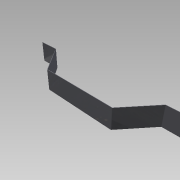
# Autodesk Inventor part: handle
Saved by Autodesk Inventor 2012 (Build 160160000, 160)
## iProperties
Created: 2012-04-18
Part Number: handle
Material: Default
Document SubType Name: Sheet Metal
Designer: thanos
Density: 1 g/cm^3
Sheet Metal Rule: Default_mm
Mass: 50.8146 g
Surface Area: 530.472 cm^2
Volume: 50.8146 cm^3
Author: thanos
Autodesk Inventor part; units mm, degrees
note: some values were not read from the file. Chosen so that the rebuilt part matches the saved one: flange form of "Plate1".
ref_plane "YZ Plane" through (0, 0, 0) normal (1, 0, 0) x (0, 1, 0)
ref_plane "XZ Plane" through (0, 0, 0) normal (0, 1, 0) x (-1, 0, 0)
ref_plane "XY Plane" through (0, 0, 0) normal (0, 0, 1) x (1, 0, 0)
sketch "Sketch3" plane through (0, 0, 0) normal (0, 0, 1) x (1, 0, 0)
  line L0 (-156.4592, 62.5093) -> (-106.4592, 62.5093)
  line L1 (-106.4592, 62.5093) -> (-39.3312, -17.4907)
  line L2 (-39.3312, -17.4907) -> (160.6688, -17.4907)
  line L3 (160.6688, -17.4907) -> (227.7967, 62.5093)
  line L4 (227.7967, 62.5093) -> (277.7967, 62.5093)
  point P0 (0, 0)
  dimension "d0" = 50
  dimension "d1" = 50
  dimension "d2" = 200
  dimension "d3" = 130
  dimension "d4" = 130
  dimension "d5" = 80
  measures "d0" distance of L0.start L0.end
  measures "d1" distance of L3.end L4.end
  measures "d2" distance of L1.end L2.end
  measures "d3" angle of L2 L1
  measures "d4" angle of L2 L3
  measures "d5" distance between parallel lines of L2 L0
contour flange "Contour Flange1" sketch "Sketch3" thickness 2 bend radius 2 width 50 along (0, 0, 1) mid plane no both sides no wall seen from (-131.4592, 62.5093, 0) lies toward (0, -1, 0) curves L0 L1 L2 L3 L4
bend "Bend1"
corner "Corner1"
equation "\"d4\" = d3"
equation "\"d6\" = BendReliefWidth"
equation "\"d7\" = BendReliefDepth"
equation "\"d8\" = MinimumRemnant"
equation "\"d9\" = BendRadius"
equation "\"d11\" = BendRadius"
equation "\"d13\" = CornerReliefSize"
equation "\"d14\" = GapSize"
equation "\"d15\" = JacobiRadiusSize"
equation "\"BendRadius\" = Thickness"
equation "\"BendReliefWidth\" = Thickness"
equation "\"BendReliefDepth\" = 0.5 * Thickness"
equation "\"CornerReliefSize\" = 4 * Thickness"
equation "\"MinimumRemnant\" = 2 * Thickness"
equation "\"TransitionRadius\" = BendRadius"
equation "\"JacobiRadiusSize\" = BendRadius"
equation "\"GapSize\" = Thickness"
equation "\"Thickness\" = 2"
body "Solid1"
